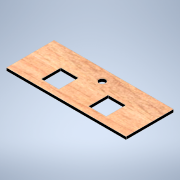
# Autodesk Inventor part: wood_front
Saved by Autodesk Inventor 2021 (Build 250183000, 183)
## iProperties
Created: 2021-08-17
Part Number: wood_front
Material: Generisch
Document SubType Name: Modeling
Designer: Tilman
Density: 1 g/cm^3
Appearance: Eloxiert - Schwarz
Author: Tilman
Autodesk Inventor part; units mm, degrees
ref_plane "YZ Plane" through (0, 0, 0) normal (1, 0, 0) x (0, 1, 0)
ref_plane "XZ Plane" through (0, 0, 0) normal (0, 1, 0) x (-1, 0, 0)
ref_plane "XY Plane" through (0, 0, 0) normal (0, 0, 1) x (1, 0, 0)
sketch "Skizze1" plane through (0, 0, 0) normal (0, 1, 0) x (-1, 0, 0)
  line L0 (0, 0) -> (-129.5, 0)
  line L1 (-129.5, 0) -> (-129.5, -51.5)
  line L2 (-129.5, -51.5) -> (0, -51.5)
  line L3 (0, -51.5) -> (0, 0)
  line L4 (-29.65, -29.2) -> (-48.65, -29.2)
  line L5 (-48.65, -29.2) -> (-48.65, -8.2)
  line L6 (-48.65, -8.2) -> (-29.65, -8.2)
  line L7 (-29.65, -8.2) -> (-29.65, -29.2)
  line L8 (-80.85, -29.2) -> (-99.85, -29.2)
  line L9 (-99.85, -29.2) -> (-99.85, -8.2)
  line L10 (-99.85, -8.2) -> (-80.85, -8.2)
  line L11 (-80.85, -8.2) -> (-80.85, -29.2)
  line L12 (-48.65, -18.7) -> (-80.85, -18.7) construction
  circle A0 centre (-64.75, -39) radius 3.5
  line L13 (-64.75, -42.5) -> (-64.75, -51.5) construction
  point P0 (-64.75, -18.7)
  point P1 (0, -25.75)
  dimension "d10" = 7
  dimension "d0" = 129.5
  dimension "d4" = 19
  dimension "d5" = 21
  dimension "d7" = 8.2
  dimension "d8" = 51.5
  dimension "d9" = 32.2
  dimension "d11" = 9
  constraints: 28 end point, 6 parallel, 5 midpoint, 3 horizontal, 3 perpendicular, 3 vertical alignment, 2 equal length, 1 point on line, 1 vertical, 2 other
  measures "d0" distance of L0.start L0.end
  measures "d4" distance of L4.start L4.end
  measures "d5" distance of L6.end L4.start
  measures "d7" distance between parallel lines of L0 L6
  measures "d8" distance of L2.end L0.start
  measures "d9" distance of L12.start L12.end
  measures "d11" distance of L13.start L13.end
extrude "Extrusion1" add sketch "Skizze1" along normal blind 3
